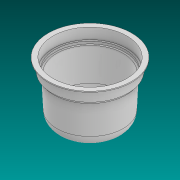
# Autodesk Inventor part: 布丁
Saved by Autodesk Inventor 2022 (Build 260153000, 153)
## iProperties
Created: 2023-03-16
Part Number: 布丁
Material: 一般
Document SubType Name: Modeling
Designer: ASUS
Density: 1 g/cm^3
Appearance: 預設
Author: ASUS
Autodesk Inventor part; units mm, degrees
ref_plane "YZ Plane" through (0, 0, 0) normal (1, 0, 0) x (0, 1, 0)
ref_plane "XZ Plane" through (0, 0, 0) normal (0, 1, 0) x (-1, 0, 0)
ref_plane "XY Plane" through (0, 0, 0) normal (0, 0, 1) x (1, 0, 0)
sketch "草圖1" plane through (0, 0, 0) normal (0, 0, 1) x (1, 0, 0)
  line L0 (0, 0) -> (-34.5, 0)
  line L1 (-34.5, 0) -> (-34.5, -0.8)
  line L2 (-34.5, -0.8) -> (0, -0.8)
  line L3 (0, -0.8) -> (0, 0)
  line L4 (0, -0.8) -> (-31.5, -0.8)
  line L5 (-31.5, -0.8) -> (-31.5, -10)
  line L6 (-31.5, -10) -> (0, -10)
  line L7 (0, -10) -> (0, -0.8)
  line L8 (0, -10) -> (-30, -10)
  line L9 (-30, -10) -> (-30, -12)
  line L10 (-30, -12) -> (0, -12)
  line L11 (0, -12) -> (0, -10)
  line L12 (-18.0931, -47) -> (0, -47)
  line L13 (0, -47) -> (0, -12)
  line L14 (0, -47) -> (-20, -47)
  line L15 (-20, -47) -> (-20, -50)
  line L16 (-20, -50) -> (0, -50)
  line L17 (0, -50) -> (0, -47)
  line L18 (0, -50) -> (-19.9, -50)
  line L19 (-19.9, -50) -> (-19.9, -55)
  line L20 (-19.9, -55) -> (0, -55)
  line L21 (0, -55) -> (0, -50)
  line L22 (0, -47) -> (-27, -47)
  line L23 (-27, -47) -> (-28.5, -12)
  dimension "d0" = 0.8
  dimension "d1" = 34.5
  dimension "d2" = 20
  dimension "d3" = 31.5
  dimension "d4" = 30
  dimension "d5" = 9.2
  dimension "d6" = 2
  dimension "d8" = 3
  dimension "d9" = 28.5
  dimension "d10" = 27
  dimension "d11" = 19.9
  dimension "d12" = 35
  dimension "d13" = 5
  constraints: 48 end point, 10 parallel, 6 perpendicular, 5 horizontal, 2 point on line, 1 collinear
  measures "d0" distance of L0.end L1.end
  measures "d1" distance of L0.start L0.end
  measures "d2" distance of L15.end L16.end
  measures "d3" distance of L5.end L6.end
  measures "d4" distance of L6.end L8.end
  measures "d5" distance of L4.end L5.end
  measures "d6" distance of L8.end L9.end
  measures "d8" distance of L14.end L15.end
  measures "d9" distance from line of L13 L23.end
  measures "d10" distance of L12.end L22.end
  measures "d11" distance of L19.end L20.end
  measures "d12" vertical distance of L22.end L23.end
  measures "d13" distance of L18.end L19.end
revolve "迴轉1" add sketch "草圖1" angle 360 about axis through (0, -47, 0) along (0, 1, 0) contours L3 L2 L1 L0 | L7 L6 L5 L2 | L11 L10 L9 L6 | L13 L12 L14 L22 L23 L10
fillet "圓角1" radius 10 1 edges at (27, -47, 0)
shell "薄殼1" thickness 1 removed faces 1 at (11.3362, 0, -5.1612)
